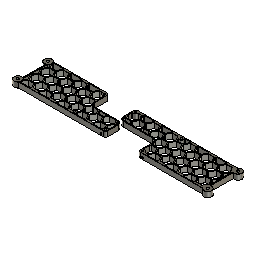
ERCF_Support_Plate_350 (Autodesk Fusion 360 design; units mm, degrees)
Autodesk Fusion 360 part; units mm, degrees
note: some values were not read from the file. Chosen so that the rebuilt part matches the saved one: which pieces of a blend or face edit are solid. Set by a fixed rule: which sketch regions a step uses.
(part 1 of 3)
sketch "Sketch1" plane through (0, 0, 0) normal (0, 0, 1) x (1, 0, 0)
  line L0 (0, 0) -> (490, 0) construction
  line L1 (490, 0) -> (490, 78) construction
  line L2 (490, 78) -> (0, 78) construction
  line L3 (0, 78) -> (0, 0) construction
  circle A0 centre (0, 78) radius 10
  circle A1 centre (0, 0) radius 10
  circle A2 centre (490, 78) radius 10
  circle A3 centre (490, 0) radius 10
  line L4 (0, 39) -> (490, 39) construction
  circle A4 centre (146, 78) radius 2.175
  circle A5 centre (146, 78) radius 6
  line L5 (0, 39) -> (23.382686, 25.5) construction
  line L6 (0, 39) -> (36.373926, 39) construction
  line L7 (23.382686, 25.5) -> (0, 12) construction
  line L8 (23.382686, 25.5) -> (42.918584, 25.5) construction
  line L9 (0, 12) -> (23.382686, -1.5) construction
  line L10 (0, 12) -> (20, 12) construction
  line L11 (220, 78) -> (220, 51.5)
  line L12 (232, 0) -> (232, 26.5)
  line L13 (152, 78) -> (152, 46.5)
  line L14 (316, 31.5) -> (316, 0)
  circle A6 centre (0, 0) radius 3
  circle A7 centre (0, 78) radius 3
  circle A8 centre (490, 0) radius 3
  circle A9 centre (490, 78) radius 3
  line L15 (8, 84) -> (146, 84)
  line L16 (226.000007, 84) -> (482, 84)
  line L17 (482, -6) -> (322.000004, -6)
  line L18 (226, -6) -> (8, -6)
  line L19 (230, 41.5) -> (306, 41.5)
  line L20 (162, 36.5) -> (222, 36.5)
  arc A10 (152, 46.5) -> (162, 36.5) centre (162, 46.5) ccw
  arc A11 (220, 51.5) -> (230, 41.5) centre (230, 51.5) ccw
  arc A12 (316, 31.5) -> (306, 41.5) centre (306, 31.5) ccw
  arc A13 (232, 26.5) -> (222, 36.5) centre (222, 26.5) ccw
  circle A14 centre (146, 0) radius 6
  circle A15 centre (146, 0) radius 2.175
  circle A16 centre (226, 78) radius 6
  circle A17 centre (226, 78) radius 2.175
  circle A18 centre (226, 0) radius 6
  circle A19 centre (226, 0) radius 2.175
  line L21 (149.5, 78) -> (149.5, 46.5)
  arc A20 (149.5, 46.5) -> (162, 34) centre (162, 46.5) ccw
  line L22 (162, 34) -> (222, 34)
  arc A21 (229.5, 26.5) -> (222, 34) centre (222, 26.5) ccw
  line L23 (229.5, 0) -> (229.5, 26.5)
  line L24 (8, 81.5) -> (146, 81.5)
  line L25 (226, -3.5) -> (8, -3.5)
  line L26 (482, -3.5) -> (322.000004, -3.5)
  line L27 (226.000007, 81.5) -> (482, 81.5)
  line L28 (6.928203, 27) -> (13.856406, 39)
  line L29 (13.856406, 39) -> (6.928203, 51)
  line L30 (6.928203, 51) -> (-6.928203, 51)
  line L31 (-6.928203, 51) -> (-13.856406, 39)
  line L32 (-13.856406, 39) -> (-6.928203, 27)
  line L33 (-6.928203, 27) -> (6.928203, 27)
  line L34 (30.310889, 13.5) -> (37.239092, 25.5)
  line L35 (37.239092, 25.5) -> (30.310889, 37.5)
  line L36 (30.310889, 37.5) -> (16.454483, 37.5)
  line L37 (16.454483, 37.5) -> (9.526279, 25.5)
  line L38 (9.526279, 25.5) -> (16.454483, 13.5)
  line L39 (16.454483, 13.5) -> (30.310889, 13.5)
  line L40 (-6.928203, 24) -> (-13.856406, 12)
  line L41 (-13.856406, 12) -> (-6.928203, 0)
  line L42 (-6.928203, 0) -> (6.928203, 0)
  line L43 (6.928203, 0) -> (13.856406, 12)
  line L44 (13.856406, 12) -> (6.928203, 24)
  line L45 (6.928203, 24) -> (-6.928203, 24)
  line L46 (16.454483, 10.5) -> (9.526279, -1.5)
  line L47 (9.526279, -1.5) -> (16.454483, -13.5)
  line L48 (16.454483, -13.5) -> (30.310889, -13.5)
  line L49 (30.310889, -13.5) -> (37.239092, -1.5)
  line L50 (37.239092, -1.5) -> (30.310889, 10.5)
  line L51 (30.310889, 10.5) -> (16.454483, 10.5)
  line L52 (6.928203, 54) -> (13.856406, 66)
  line L53 (13.856406, 66) -> (6.928203, 78)
  line L54 (6.928203, 78) -> (-6.928203, 78)
  line L55 (-6.928203, 78) -> (-13.856406, 66)
  line L56 (-13.856406, 66) -> (-6.928203, 54)
  line L57 (-6.928203, 54) -> (6.928203, 54)
  line L58 (3, 78) -> (3, 0)
  line L59 (487, 78) -> (487, 0)
  line L60 (484, 78) -> (484, 0)
  line L61 (6, 78) -> (6, 0)
  line L62 (222.5, 78) -> (222.5, 51.5)
  arc A22 (222.5, 51.5) -> (230, 44) centre (230, 51.5) ccw
  line L63 (230, 44) -> (306, 44)
  arc A23 (318.5, 31.5) -> (306, 44) centre (306, 31.5) ccw
  line L64 (318.5, 31.5) -> (318.5, 0)
  circle A24 centre (344, 78) radius 2.175
  circle A25 centre (344, 78) radius 6
  circle A26 centre (322, 0) radius 2.175
  circle A27 centre (322, 0) radius 6
  line L65 (32.908965, 12) -> (39.837169, 0)
  line L66 (39.837169, 24) -> (32.908965, 12)
  line L67 (53.693575, 24) -> (39.837169, 24)
  line L68 (60.621778, 12) -> (53.693575, 24)
  line L69 (53.693575, 0) -> (60.621778, 12)
  line L70 (63.219854, 10.5) -> (56.291651, -1.5)
  line L71 (39.837169, 0) -> (53.693575, 0)
  line L72 (53.693575, -3) -> (39.837169, -3)
  line L73 (60.621778, -15) -> (53.693575, -3)
  line L74 (53.693575, -27) -> (60.621778, -15)
  line L75 (39.837169, -27) -> (53.693575, -27)
  line L76 (32.908965, -15) -> (39.837169, -27)
  line L77 (39.837169, -3) -> (32.908965, -15)
  line L78 (77.076261, 10.5) -> (63.219854, 10.5)
  line L79 (56.291651, -1.5) -> (63.219854, -13.5)
  line L80 (63.219854, -13.5) -> (77.076261, -13.5)
  line L81 (77.076261, -13.5) -> (84.004464, -1.5)
  line L82 (84.004464, -1.5) -> (77.076261, 10.5)
  line L83 (77.076261, -16.5) -> (63.219854, -16.5)
  line L84 (63.219854, -16.5) -> (56.291651, -28.5)
  line L85 (56.291651, -28.5) -> (63.219854, -40.5)
  line L86 (63.219854, -40.5) -> (77.076261, -40.5)
  line L87 (77.076261, -40.5) -> (84.004464, -28.5)
  line L88 (84.004464, -28.5) -> (77.076261, -16.5)
  line L89 (79.674337, -15) -> (86.60254, -27)
  line L90 (86.60254, -3) -> (79.674337, -15)
  line L91 (100.458947, -3) -> (86.60254, -3)
  line L92 (107.38715, -15) -> (100.458947, -3)
  line L93 (100.458947, -27) -> (107.38715, -15)
  line L94 (109.985226, -16.5) -> (103.057023, -28.5)
  line L95 (86.60254, -27) -> (100.458947, -27)
  line L96 (100.458947, -30) -> (86.60254, -30)
  line L97 (107.38715, -42) -> (100.458947, -30)
  line L98 (100.458947, -54) -> (107.38715, -42)
  line L99 (86.60254, -54) -> (100.458947, -54)
  line L100 (79.674337, -42) -> (86.60254, -54)
  line L101 (86.60254, -30) -> (79.674337, -42)
  line L102 (123.841633, -16.5) -> (109.985226, -16.5)
  line L103 (103.057023, -28.5) -> (109.985226, -40.5)
  line L104 (109.985226, -40.5) -> (123.841633, -40.5)
  line L105 (123.841633, -40.5) -> (130.769836, -28.5)
  line L106 (130.769836, -28.5) -> (123.841633, -16.5)
  line L107 (123.841633, -43.5) -> (109.985226, -43.5)
  line L108 (109.985226, -43.5) -> (103.057023, -55.5)
  line L109 (103.057023, -55.5) -> (109.985226, -67.5)
  line L110 (109.985226, -67.5) -> (123.841633, -67.5)
  line L111 (123.841633, -67.5) -> (130.769836, -55.5)
  line L112 (130.769836, -55.5) -> (123.841633, -43.5)
  line L113 (126.439709, -42) -> (133.367912, -54)
  line L114 (133.367912, -30) -> (126.439709, -42)
  line L115 (147.224319, -30) -> (133.367912, -30)
  line L116 (154.152522, -42) -> (147.224319, -30)
  line L117 (147.224319, -54) -> (154.152522, -42)
  line L118 (156.750598, -43.5) -> (149.822395, -55.5)
  line L119 (133.367912, -54) -> (147.224319, -54)
  line L120 (147.224319, -57) -> (133.367912, -57)
  line L121 (154.152522, -69) -> (147.224319, -57)
  line L122 (147.224319, -81) -> (154.152522, -69)
  line L123 (133.367912, -81) -> (147.224319, -81)
  line L124 (126.439709, -69) -> (133.367912, -81)
  line L125 (133.367912, -57) -> (126.439709, -69)
  line L126 (170.607005, -43.5) -> (156.750598, -43.5)
  line L127 (149.822395, -55.5) -> (156.750598, -67.5)
  line L128 (156.750598, -67.5) -> (170.607005, -67.5)
  line L129 (170.607005, -67.5) -> (177.535208, -55.5)
  line L130 (177.535208, -55.5) -> (170.607005, -43.5)
  line L131 (170.607005, -70.5) -> (156.750598, -70.5)
  line L132 (156.750598, -70.5) -> (149.822395, -82.5)
  line L133 (149.822395, -82.5) -> (156.750598, -94.5)
  line L134 (156.750598, -94.5) -> (170.607005, -94.5)
  line L135 (170.607005, -94.5) -> (177.535208, -82.5)
  line L136 (177.535208, -82.5) -> (170.607005, -70.5)
  line L137 (173.205081, -69) -> (180.133284, -81)
  line L138 (180.133284, -57) -> (173.205081, -69)
  line L139 (193.98969, -57) -> (180.133284, -57)
  line L140 (200.917894, -69) -> (193.98969, -57)
  line L141 (193.98969, -81) -> (200.917894, -69)
  line L142 (203.51597, -70.5) -> (196.587767, -82.5)
  line L143 (180.133284, -81) -> (193.98969, -81)
  line L144 (193.98969, -84) -> (180.133284, -84)
  line L145 (200.917894, -96) -> (193.98969, -84)
  line L146 (193.98969, -108) -> (200.917894, -96)
  line L147 (180.133284, -108) -> (193.98969, -108)
  line L148 (173.205081, -96) -> (180.133284, -108)
  line L149 (180.133284, -84) -> (173.205081, -96)
  line L150 (217.372376, -70.5) -> (203.51597, -70.5)
  line L151 (196.587767, -82.5) -> (203.51597, -94.5)
  line L152 (203.51597, -94.5) -> (217.372376, -94.5)
  line L153 (217.372376, -94.5) -> (224.30058, -82.5)
  line L154 (224.30058, -82.5) -> (217.372376, -70.5)
  line L155 (217.372376, -97.5) -> (203.51597, -97.5)
  line L156 (203.51597, -97.5) -> (196.587767, -109.5)
  line L157 (196.587767, -109.5) -> (203.51597, -121.5)
  line L158 (203.51597, -121.5) -> (217.372376, -121.5)
  line L159 (217.372376, -121.5) -> (224.30058, -109.5)
  line L160 (224.30058, -109.5) -> (217.372376, -97.5)
  line L161 (219.970453, -96) -> (226.898656, -108)
  line L162 (226.898656, -84) -> (219.970453, -96)
  line L163 (240.755062, -84) -> (226.898656, -84)
  line L164 (247.683265, -96) -> (240.755062, -84)
  line L165 (240.755062, -108) -> (247.683265, -96)
  line L166 (250.281342, -97.5) -> (243.353138, -109.5)
  line L167 (226.898656, -108) -> (240.755062, -108)
  line L168 (240.755062, -111) -> (226.898656, -111)
  line L169 (247.683265, -123) -> (240.755062, -111)
  line L170 (240.755062, -135) -> (247.683265, -123)
  line L171 (226.898656, -135) -> (240.755062, -135)
  line L172 (219.970453, -123) -> (226.898656, -135)
  line L173 (226.898656, -111) -> (219.970453, -123)
  line L174 (264.137748, -97.5) -> (250.281342, -97.5)
  line L175 (243.353138, -109.5) -> (250.281342, -121.5)
  line L176 (250.281342, -121.5) -> (264.137748, -121.5)
  line L177 (264.137748, -121.5) -> (271.065951, -109.5)
  line L178 (271.065951, -109.5) -> (264.137748, -97.5)
  line L179 (264.137748, -124.5) -> (250.281342, -124.5)
  line L180 (250.281342, -124.5) -> (243.353138, -136.5)
  line L181 (243.353138, -136.5) -> (250.281342, -148.5)
  line L182 (250.281342, -148.5) -> (264.137748, -148.5)
  line L183 (264.137748, -148.5) -> (271.065951, -136.5)
  line L184 (271.065951, -136.5) -> (264.137748, -124.5)
  line L185 (266.735824, -123) -> (273.664028, -135)
  line L186 (273.664028, -111) -> (266.735824, -123)
  line L187 (287.520434, -111) -> (273.664028, -111)
  line L188 (294.448637, -123) -> (287.520434, -111)
  line L189 (287.520434, -135) -> (294.448637, -123)
  line L190 (297.046713, -124.5) -> (290.11851, -136.5)
  line L191 (273.664028, -135) -> (287.520434, -135)
  line L192 (287.520434, -138) -> (273.664028, -138)
  line L193 (294.448637, -150) -> (287.520434, -138)
  line L194 (287.520434, -162) -> (294.448637, -150)
  line L195 (273.664028, -162) -> (287.520434, -162)
  line L196 (266.735824, -150) -> (273.664028, -162)
  line L197 (273.664028, -138) -> (266.735824, -150)
  line L198 (310.90312, -124.5) -> (297.046713, -124.5)
  line L199 (290.11851, -136.5) -> (297.046713, -148.5)
  line L200 (297.046713, -148.5) -> (310.90312, -148.5)
  line L201 (310.90312, -148.5) -> (317.831323, -136.5)
  line L202 (317.831323, -136.5) -> (310.90312, -124.5)
  line L203 (310.90312, -151.5) -> (297.046713, -151.5)
  line L204 (297.046713, -151.5) -> (290.11851, -163.5)
  line L205 (290.11851, -163.5) -> (297.046713, -175.5)
  line L206 (297.046713, -175.5) -> (310.90312, -175.5)
  line L207 (310.90312, -175.5) -> (317.831323, -163.5)
  line L208 (317.831323, -163.5) -> (310.90312, -151.5)
  line L209 (313.501196, -150) -> (320.429399, -162)
  line L210 (320.429399, -138) -> (313.501196, -150)
  line L211 (334.285806, -138) -> (320.429399, -138)
  line L212 (341.214009, -150) -> (334.285806, -138)
  line L213 (334.285806, -162) -> (341.214009, -150)
  line L214 (343.812085, -151.5) -> (336.883882, -163.5)
  line L215 (320.429399, -162) -> (334.285806, -162)
  line L216 (334.285806, -165) -> (320.429399, -165)
  line L217 (341.214009, -177) -> (334.285806, -165)
  line L218 (334.285806, -189) -> (341.214009, -177)
  line L219 (320.429399, -189) -> (334.285806, -189)
  line L220 (313.501196, -177) -> (320.429399, -189)
  line L221 (320.429399, -165) -> (313.501196, -177)
  line L222 (357.668492, -151.5) -> (343.812085, -151.5)
  line L223 (336.883882, -163.5) -> (343.812085, -175.5)
  line L224 (343.812085, -175.5) -> (357.668492, -175.5)
  line L225 (357.668492, -175.5) -> (364.596695, -163.5)
  line L226 (364.596695, -163.5) -> (357.668492, -151.5)
  line L227 (357.668492, -178.5) -> (343.812085, -178.5)
  line L228 (343.812085, -178.5) -> (336.883882, -190.5)
  line L229 (336.883882, -190.5) -> (343.812085, -202.5)
  line L230 (343.812085, -202.5) -> (357.668492, -202.5)
  line L231 (357.668492, -202.5) -> (364.596695, -190.5)
  line L232 (364.596695, -190.5) -> (357.668492, -178.5)
  line L233 (360.266568, -177) -> (367.194771, -189)
  line L234 (367.194771, -165) -> (360.266568, -177)
  line L235 (381.051178, -165) -> (367.194771, -165)
  line L236 (387.979381, -177) -> (381.051178, -165)
  line L237 (381.051178, -189) -> (387.979381, -177)
  line L238 (390.577457, -178.5) -> (383.649254, -190.5)
  line L239 (367.194771, -189) -> (381.051178, -189)
  line L240 (381.051178, -192) -> (367.194771, -192)
  line L241 (387.979381, -204) -> (381.051178, -192)
  line L242 (381.051178, -216) -> (387.979381, -204)
  line L243 (367.194771, -216) -> (381.051178, -216)
  line L244 (360.266568, -204) -> (367.194771, -216)
  line L245 (367.194771, -192) -> (360.266568, -204)
  line L246 (404.433864, -178.5) -> (390.577457, -178.5)
  line L247 (383.649254, -190.5) -> (390.577457, -202.5)
  line L248 (390.577457, -202.5) -> (404.433864, -202.5)
  line L249 (404.433864, -202.5) -> (411.362067, -190.5)
  line L250 (411.362067, -190.5) -> (404.433864, -178.5)
  line L251 (404.433864, -205.5) -> (390.577457, -205.5)
  line L252 (390.577457, -205.5) -> (383.649254, -217.5)
  line L253 (383.649254, -217.5) -> (390.577457, -229.5)
  line L254 (390.577457, -229.5) -> (404.433864, -229.5)
  line L255 (404.433864, -229.5) -> (411.362067, -217.5)
  line L256 (411.362067, -217.5) -> (404.433864, -205.5)
  line L257 (9.523594, 79.495348) -> (16.451797, 67.495348)
  line L258 (16.451797, 91.495348) -> (9.523594, 79.495348)
  line L259 (30.308203, 91.495348) -> (16.451797, 91.495348)
  line L260 (37.236406, 79.495348) -> (30.308203, 91.495348)
  line L261 (30.308203, 67.495348) -> (37.236406, 79.495348)
  line L262 (39.834483, 77.995348) -> (32.906279, 65.995348)
  line L263 (16.451797, 67.495348) -> (30.308203, 67.495348)
  line L264 (30.308203, 64.495348) -> (16.451797, 64.495348)
  line L265 (37.236406, 52.495348) -> (30.308203, 64.495348)
  line L266 (30.308203, 40.495348) -> (37.236406, 52.495348)
  line L267 (16.451797, 40.495348) -> (30.308203, 40.495348)
  line L268 (9.523594, 52.495348) -> (16.451797, 40.495348)
  line L269 (16.451797, 64.495348) -> (9.523594, 52.495348)
  line L270 (53.690889, 77.995348) -> (39.834483, 77.995348)
  line L271 (32.906279, 65.995348) -> (39.834483, 53.995348)
  line L272 (39.834483, 53.995348) -> (53.690889, 53.995348)
  line L273 (53.690889, 53.995348) -> (60.619092, 65.995348)
  line L274 (60.619092, 65.995348) -> (53.690889, 77.995348)
  line L275 (53.690889, 50.995348) -> (39.834483, 50.995348)
  line L276 (39.834483, 50.995348) -> (32.906279, 38.995348)
  line L277 (32.906279, 38.995348) -> (39.834483, 26.995348)
  line L278 (39.834483, 26.995348) -> (53.690889, 26.995348)
  line L279 (53.690889, 26.995348) -> (60.619092, 38.995348)
  line L280 (60.619092, 38.995348) -> (53.690889, 50.995348)
  line L281 (56.288965, 52.495348) -> (63.217169, 40.495348)
  line L282 (63.217169, 64.495348) -> (56.288965, 52.495348)
  line L283 (77.073575, 64.495348) -> (63.217169, 64.495348)
  line L284 (84.001778, 52.495348) -> (77.073575, 64.495348)
  line L285 (77.073575, 40.495348) -> (84.001778, 52.495348)
  line L286 (86.599854, 50.995348) -> (79.671651, 38.995348)
  line L287 (63.217169, 40.495348) -> (77.073575, 40.495348)
  line L288 (77.073575, 37.495348) -> (63.217169, 37.495348)
  line L289 (84.001778, 25.495348) -> (77.073575, 37.495348)
  line L290 (77.073575, 13.495348) -> (84.001778, 25.495348)
  line L291 (63.217169, 13.495348) -> (77.073575, 13.495348)
  line L292 (56.288965, 25.495348) -> (63.217169, 13.495348)
  line L293 (63.217169, 37.495348) -> (56.288965, 25.495348)
  line L294 (100.456261, 50.995348) -> (86.599854, 50.995348)
  line L295 (79.671651, 38.995348) -> (86.599854, 26.995348)
  line L296 (86.599854, 26.995348) -> (100.456261, 26.995348)
  line L297 (100.456261, 26.995348) -> (107.384464, 38.995348)
  line L298 (107.384464, 38.995348) -> (100.456261, 50.995348)
  line L299 (100.456261, 23.995348) -> (86.599854, 23.995348)
  line L300 (86.599854, 23.995348) -> (79.671651, 11.995348)
  line L301 (79.671651, 11.995348) -> (86.599854, -0.004652)
  line L302 (86.599854, -0.004652) -> (100.456261, -0.004652)
  line L303 (100.456261, -0.004652) -> (107.384464, 11.995348)
  line L304 (107.384464, 11.995348) -> (100.456261, 23.995348)
  line L305 (103.054337, 25.495348) -> (109.98254, 13.495348)
  line L306 (109.98254, 37.495348) -> (103.054337, 25.495348)
  line L307 (123.838947, 37.495348) -> (109.98254, 37.495348)
  line L308 (130.76715, 25.495348) -> (123.838947, 37.495348)
  line L309 (123.838947, 13.495348) -> (130.76715, 25.495348)
  line L310 (133.365226, 23.995348) -> (126.437023, 11.995348)
  line L311 (109.98254, 13.495348) -> (123.838947, 13.495348)
  line L312 (123.838947, 10.495348) -> (109.98254, 10.495348)
  line L313 (130.76715, -1.504652) -> (123.838947, 10.495348)
  line L314 (123.838947, -13.504652) -> (130.76715, -1.504652)
  line L315 (109.98254, -13.504652) -> (123.838947, -13.504652)
  line L316 (103.054337, -1.504652) -> (109.98254, -13.504652)
  line L317 (109.98254, 10.495348) -> (103.054337, -1.504652)
  line L318 (147.221633, 23.995348) -> (133.365226, 23.995348)
  line L319 (126.437023, 11.995348) -> (133.365226, -0.004652)
  line L320 (133.365226, -0.004652) -> (147.221633, -0.004652)
  line L321 (147.221633, -0.004652) -> (154.149836, 11.995348)
  line L322 (154.149836, 11.995348) -> (147.221633, 23.995348)
  line L323 (147.221633, -3.004652) -> (133.365226, -3.004652)
  line L324 (133.365226, -3.004652) -> (126.437023, -15.004652)
  line L325 (126.437023, -15.004652) -> (133.365226, -27.004652)
  line L326 (133.365226, -27.004652) -> (147.221633, -27.004652)
  line L327 (147.221633, -27.004652) -> (154.149836, -15.004652)
  line L328 (154.149836, -15.004652) -> (147.221633, -3.004652)
  line L329 (149.819709, -1.504652) -> (156.747912, -13.504652)
  line L330 (156.747912, 10.495348) -> (149.819709, -1.504652)
  line L331 (170.604319, 10.495348) -> (156.747912, 10.495348)
  line L332 (177.532522, -1.504652) -> (170.604319, 10.495348)
  line L333 (170.604319, -13.504652) -> (177.532522, -1.504652)
  line L334 (180.130598, -3.004652) -> (173.202395, -15.004652)
  line L335 (156.747912, -13.504652) -> (170.604319, -13.504652)
  line L336 (170.604319, -16.504652) -> (156.747912, -16.504652)
  line L337 (177.532522, -28.504652) -> (170.604319, -16.504652)
  line L338 (170.604319, -40.504652) -> (177.532522, -28.504652)
  line L339 (156.747912, -40.504652) -> (170.604319, -40.504652)
  line L340 (149.819709, -28.504652) -> (156.747912, -40.504652)
  line L341 (156.747912, -16.504652) -> (149.819709, -28.504652)
  line L342 (193.987005, -3.004652) -> (180.130598, -3.004652)
  line L343 (173.202395, -15.004652) -> (180.130598, -27.004652)
  line L344 (180.130598, -27.004652) -> (193.987005, -27.004652)
  line L345 (193.987005, -27.004652) -> (200.915208, -15.004652)
  line L346 (200.915208, -15.004652) -> (193.987005, -3.004652)
  line L347 (193.987005, -30.004652) -> (180.130598, -30.004652)
  line L348 (180.130598, -30.004652) -> (173.202395, -42.004652)
  line L349 (173.202395, -42.004652) -> (180.130598, -54.004652)
  line L350 (180.130598, -54.004652) -> (193.987005, -54.004652)
  line L351 (193.987005, -54.004652) -> (200.915208, -42.004652)
  line L352 (200.915208, -42.004652) -> (193.987005, -30.004652)
  line L353 (196.585081, -28.504652) -> (203.513284, -40.504652)
  line L354 (203.513284, -16.504652) -> (196.585081, -28.504652)
  line L355 (217.36969, -16.504652) -> (203.513284, -16.504652)
  line L356 (224.297894, -28.504652) -> (217.36969, -16.504652)
  line L357 (217.36969, -40.504652) -> (224.297894, -28.504652)
  line L358 (226.89597, -30.004652) -> (219.967767, -42.004652)
  line L359 (203.513284, -40.504652) -> (217.36969, -40.504652)
  line L360 (217.36969, -43.504652) -> (203.513284, -43.504652)
  line L361 (224.297894, -55.504652) -> (217.36969, -43.504652)
  line L362 (217.36969, -67.504652) -> (224.297894, -55.504652)
  line L363 (203.513284, -67.504652) -> (217.36969, -67.504652)
  line L364 (196.585081, -55.504652) -> (203.513284, -67.504652)
  line L365 (203.513284, -43.504652) -> (196.585081, -55.504652)
  line L366 (240.752376, -30.004652) -> (226.89597, -30.004652)
  line L367 (219.967767, -42.004652) -> (226.89597, -54.004652)
  line L368 (226.89597, -54.004652) -> (240.752376, -54.004652)
  line L369 (240.752376, -54.004652) -> (247.68058, -42.004652)
  line L370 (247.68058, -42.004652) -> (240.752376, -30.004652)
  line L371 (240.752376, -57.004652) -> (226.89597, -57.004652)
  line L372 (226.89597, -57.004652) -> (219.967767, -69.004652)
  line L373 (219.967767, -69.004652) -> (226.89597, -81.004652)
  line L374 (226.89597, -81.004652) -> (240.752376, -81.004652)
  line L375 (240.752376, -81.004652) -> (247.68058, -69.004652)
  line L376 (247.68058, -69.004652) -> (240.752376, -57.004652)
  line L377 (243.350453, -55.504652) -> (250.278656, -67.504652)
  line L378 (250.278656, -43.504652) -> (243.350453, -55.504652)
  line L379 (264.135062, -43.504652) -> (250.278656, -43.504652)
  line L380 (271.063265, -55.504652) -> (264.135062, -43.504652)
  line L381 (264.135062, -67.504652) -> (271.063265, -55.504652)
  line L382 (273.661342, -57.004652) -> (266.733138, -69.004652)
  line L383 (250.278656, -67.504652) -> (264.135062, -67.504652)
  line L384 (264.135062, -70.504652) -> (250.278656, -70.504652)
  line L385 (271.063265, -82.504652) -> (264.135062, -70.504652)
  line L386 (264.135062, -94.504652) -> (271.063265, -82.504652)
  line L387 (250.278656, -94.504652) -> (264.135062, -94.504652)
  line L388 (243.350453, -82.504652) -> (250.278656, -94.504652)
  line L389 (250.278656, -70.504652) -> (243.350453, -82.504652)
  line L390 (287.517748, -57.004652) -> (273.661342, -57.004652)
  line L391 (266.733138, -69.004652) -> (273.661342, -81.004652)
  line L392 (273.661342, -81.004652) -> (287.517748, -81.004652)
  line L393 (287.517748, -81.004652) -> (294.445951, -69.004652)
  line L394 (294.445951, -69.004652) -> (287.517748, -57.004652)
  line L395 (287.517748, -84.004652) -> (273.661342, -84.004652)
  line L396 (273.661342, -84.004652) -> (266.733138, -96.004652)
  line L397 (266.733138, -96.004652) -> (273.661342, -108.004652)
  line L398 (273.661342, -108.004652) -> (287.517748, -108.004652)
  line L399 (287.517748, -108.004652) -> (294.445951, -96.004652)
  line L400 (294.445951, -96.004652) -> (287.517748, -84.004652)
  line L401 (290.115824, -82.504652) -> (297.044028, -94.504652)
  line L402 (297.044028, -70.504652) -> (290.115824, -82.504652)
  line L403 (310.900434, -70.504652) -> (297.044028, -70.504652)
  line L404 (317.828637, -82.504652) -> (310.900434, -70.504652)
  line L405 (310.900434, -94.504652) -> (317.828637, -82.504652)
  line L406 (320.426713, -84.004652) -> (313.49851, -96.004652)
  line L407 (297.044028, -94.504652) -> (310.900434, -94.504652)
  line L408 (310.900434, -97.504652) -> (297.044028, -97.504652)
  line L409 (317.828637, -109.504652) -> (310.900434, -97.504652)
  line L410 (310.900434, -121.504652) -> (317.828637, -109.504652)
  line L411 (297.044028, -121.504652) -> (310.900434, -121.504652)
  line L412 (290.115824, -109.504652) -> (297.044028, -121.504652)
  line L413 (297.044028, -97.504652) -> (290.115824, -109.504652)
  line L414 (334.28312, -84.004652) -> (320.426713, -84.004652)
  line L415 (313.49851, -96.004652) -> (320.426713, -108.004652)
  line L416 (320.426713, -108.004652) -> (334.28312, -108.004652)
  line L417 (334.28312, -108.004652) -> (341.211323, -96.004652)
  line L418 (341.211323, -96.004652) -> (334.28312, -84.004652)
  line L419 (334.28312, -111.004652) -> (320.426713, -111.004652)
  line L420 (320.426713, -111.004652) -> (313.49851, -123.004652)
  line L421 (313.49851, -123.004652) -> (320.426713, -135.004652)
  line L422 (320.426713, -135.004652) -> (334.28312, -135.004652)
  line L423 (334.28312, -135.004652) -> (341.211323, -123.004652)
  line L424 (341.211323, -123.004652) -> (334.28312, -111.004652)
  line L425 (336.881196, -109.504652) -> (343.809399, -121.504652)
  line L426 (343.809399, -97.504652) -> (336.881196, -109.504652)
  line L427 (357.665806, -97.504652) -> (343.809399, -97.504652)
  line L428 (364.594009, -109.504652) -> (357.665806, -97.504652)
  line L429 (357.665806, -121.504652) -> (364.594009, -109.504652)
  line L430 (367.192085, -111.004652) -> (360.263882, -123.004652)
  line L431 (343.809399, -121.504652) -> (357.665806, -121.504652)
  line L432 (357.665806, -124.504652) -> (343.809399, -124.504652)
  line L433 (364.594009, -136.504652) -> (357.665806, -124.504652)
  line L434 (357.665806, -148.504652) -> (364.594009, -136.504652)
  line L435 (343.809399, -148.504652) -> (357.665806, -148.504652)
  line L436 (336.881196, -136.504652) -> (343.809399, -148.504652)
  line L437 (343.809399, -124.504652) -> (336.881196, -136.504652)
  line L438 (381.048492, -111.004652) -> (367.192085, -111.004652)
  line L439 (360.263882, -123.004652) -> (367.192085, -135.004652)
  line L440 (367.192085, -135.004652) -> (381.048492, -135.004652)
  line L441 (381.048492, -135.004652) -> (387.976695, -123.004652)
  line L442 (387.976695, -123.004652) -> (381.048492, -111.004652)
  line L443 (381.048492, -138.004652) -> (367.192085, -138.004652)
  line L444 (367.192085, -138.004652) -> (360.263882, -150.004652)
  line L445 (360.263882, -150.004652) -> (367.192085, -162.004652)
  line L446 (367.192085, -162.004652) -> (381.048492, -162.004652)
  line L447 (381.048492, -162.004652) -> (387.976695, -150.004652)
  line L448 (387.976695, -150.004652) -> (381.048492, -138.004652)
  line L449 (383.646568, -136.504652) -> (390.574771, -148.504652)
  line L450 (390.574771, -124.504652) -> (383.646568, -136.504652)
  line L451 (404.431178, -124.504652) -> (390.574771, -124.504652)
  line L452 (411.359381, -136.504652) -> (404.431178, -124.504652)
  line L453 (404.431178, -148.504652) -> (411.359381, -136.504652)
  line L454 (413.957457, -138.004652) -> (407.029254, -150.004652)
  line L455 (390.574771, -148.504652) -> (404.431178, -148.504652)
  line L456 (404.431178, -151.504652) -> (390.574771, -151.504652)
  line L457 (411.359381, -163.504652) -> (404.431178, -151.504652)
  line L458 (404.431178, -175.504652) -> (411.359381, -163.504652)
  line L459 (390.574771, -175.504652) -> (404.431178, -175.504652)
  line L460 (383.646568, -163.504652) -> (390.574771, -175.504652)
  line L461 (390.574771, -151.504652) -> (383.646568, -163.504652)
  line L462 (427.813864, -138.004652) -> (413.957457, -138.004652)
  line L463 (407.029254, -150.004652) -> (413.957457, -162.004652)
  line L464 (413.957457, -162.004652) -> (427.813864, -162.004652)
  line L465 (427.813864, -162.004652) -> (434.742067, -150.004652)
  line L466 (434.742067, -150.004652) -> (427.813864, -138.004652)
  line L467 (427.813864, -165.004652) -> (413.957457, -165.004652)
  line L468 (413.957457, -165.004652) -> (407.029254, -177.004652)
  line L469 (407.029254, -177.004652) -> (413.957457, -189.004652)
  line L470 (413.957457, -189.004652) -> (427.813864, -189.004652)
  line L471 (427.813864, -189.004652) -> (434.742067, -177.004652)
  line L472 (434.742067, -177.004652) -> (427.813864, -165.004652)
  line L473 (32.903594, 119.990696) -> (39.831797, 107.990696)
  line L474 (39.831797, 131.990696) -> (32.903594, 119.990696)
  line L475 (53.688203, 131.990696) -> (39.831797, 131.990696)
  line L476 (60.616406, 119.990696) -> (53.688203, 131.990696)
  line L477 (53.688203, 107.990696) -> (60.616406, 119.990696)
  line L478 (63.214483, 118.490696) -> (56.286279, 106.490696)
  line L479 (39.831797, 107.990696) -> (53.688203, 107.990696)
  line L480 (53.688203, 104.990696) -> (39.831797, 104.990696)
  line L481 (60.616406, 92.990696) -> (53.688203, 104.990696)
  line L482 (53.688203, 80.990696) -> (60.616406, 92.990696)
  line L483 (39.831797, 80.990696) -> (53.688203, 80.990696)
  line L484 (32.903594, 92.990696) -> (39.831797, 80.990696)
  line L485 (39.831797, 104.990696) -> (32.903594, 92.990696)
  line L486 (77.070889, 118.490696) -> (63.214483, 118.490696)
  line L487 (56.286279, 106.490696) -> (63.214483, 94.490696)
  line L488 (63.214483, 94.490696) -> (77.070889, 94.490696)
  line L489 (77.070889, 94.490696) -> (83.999092, 106.490696)
  line L490 (83.999092, 106.490696) -> (77.070889, 118.490696)
  line L491 (77.070889, 91.490696) -> (63.214483, 91.490696)
  line L492 (63.214483, 91.490696) -> (56.286279, 79.490696)
  line L493 (56.286279, 79.490696) -> (63.214483, 67.490696)
  line L494 (63.214483, 67.490696) -> (77.070889, 67.490696)
  line L495 (77.070889, 67.490696) -> (83.999092, 79.490696)
  line L496 (83.999092, 79.490696) -> (77.070889, 91.490696)
  line L497 (79.668965, 92.990696) -> (86.597169, 80.990696)
  line L498 (86.597169, 104.990696) -> (79.668965, 92.990696)
  line L499 (100.453575, 104.990696) -> (86.597169, 104.990696)
  line L500 (107.381778, 92.990696) -> (100.453575, 104.990696)
  line L501 (100.453575, 80.990696) -> (107.381778, 92.990696)
  line L502 (109.979854, 91.490696) -> (103.051651, 79.490696)
  line L503 (86.597169, 80.990696) -> (100.453575, 80.990696)
  line L504 (100.453575, 77.990696) -> (86.597169, 77.990696)
  line L505 (107.381778, 65.990696) -> (100.453575, 77.990696)
  line L506 (100.453575, 53.990696) -> (107.381778, 65.990696)
  line L507 (86.597169, 53.990696) -> (100.453575, 53.990696)
  line L508 (79.668965, 65.990696) -> (86.597169, 53.990696)
  line L509 (86.597169, 77.990696) -> (79.668965, 65.990696)
  line L510 (123.836261, 91.490696) -> (109.979854, 91.490696)
  line L511 (103.051651, 79.490696) -> (109.979854, 67.490696)
  line L512 (109.979854, 67.490696) -> (123.836261, 67.490696)
  line L513 (123.836261, 67.490696) -> (130.764464, 79.490696)
  line L514 (130.764464, 79.490696) -> (123.836261, 91.490696)
  line L515 (123.836261, 64.490696) -> (109.979854, 64.490696)
  line L516 (109.979854, 64.490696) -> (103.051651, 52.490696)
  line L517 (103.051651, 52.490696) -> (109.979854, 40.490696)
  line L518 (109.979854, 40.490696) -> (123.836261, 40.490696)
  line L519 (123.836261, 40.490696) -> (130.764464, 52.490696)
  line L520 (130.764464, 52.490696) -> (123.836261, 64.490696)
  line L521 (126.434337, 65.990696) -> (133.36254, 53.990696)
  line L522 (133.36254, 77.990696) -> (126.434337, 65.990696)
  line L523 (147.218947, 77.990696) -> (133.36254, 77.990696)
  line L524 (154.14715, 65.990696) -> (147.218947, 77.990696)
  line L525 (147.218947, 53.990696) -> (154.14715, 65.990696)
  line L526 (156.745226, 64.490696) -> (149.817023, 52.490696)
  line L527 (133.36254, 53.990696) -> (147.218947, 53.990696)
  line L528 (147.218947, 50.990696) -> (133.36254, 50.990696)
  line L529 (154.14715, 38.990696) -> (147.218947, 50.990696)
  line L530 (147.218947, 26.990696) -> (154.14715, 38.990696)
  line L531 (133.36254, 26.990696) -> (147.218947, 26.990696)
  line L532 (126.434337, 38.990696) -> (133.36254, 26.990696)
  line L533 (133.36254, 50.990696) -> (126.434337, 38.990696)
  line L534 (170.601633, 64.490696) -> (156.745226, 64.490696)
  line L535 (149.817023, 52.490696) -> (156.745226, 40.490696)
  line L536 (156.745226, 40.490696) -> (170.601633, 40.490696)
  line L537 (170.601633, 40.490696) -> (177.529836, 52.490696)
  line L538 (177.529836, 52.490696) -> (170.601633, 64.490696)
  line L539 (170.601633, 37.490696) -> (156.745226, 37.490696)
  line L540 (156.745226, 37.490696) -> (149.817023, 25.490696)
  line L541 (149.817023, 25.490696) -> (156.745226, 13.490696)
  line L542 (156.745226, 13.490696) -> (170.601633, 13.490696)
  line L543 (170.601633, 13.490696) -> (177.529836, 25.490696)
  line L544 (177.529836, 25.490696) -> (170.601633, 37.490696)
  line L545 (173.199709, 38.990696) -> (180.127912, 26.990696)
  line L546 (180.127912, 50.990696) -> (173.199709, 38.990696)
  line L547 (193.984319, 50.990696) -> (180.127912, 50.990696)
  line L548 (200.912522, 38.990696) -> (193.984319, 50.990696)
  line L549 (193.984319, 26.990696) -> (200.912522, 38.990696)
  line L550 (203.510598, 37.490696) -> (196.582395, 25.490696)
  line L551 (180.127912, 26.990696) -> (193.984319, 26.990696)
  line L552 (193.984319, 23.990696) -> (180.127912, 23.990696)
  line L553 (200.912522, 11.990696) -> (193.984319, 23.990696)
  line L554 (193.984319, -0.009304) -> (200.912522, 11.990696)
  line L555 (180.127912, -0.009304) -> (193.984319, -0.009304)
  line L556 (173.199709, 11.990696) -> (180.127912, -0.009304)
  line L557 (180.127912, 23.990696) -> (173.199709, 11.990696)
  line L558 (217.367005, 37.490696) -> (203.510598, 37.490696)
  line L559 (196.582395, 25.490696) -> (203.510598, 13.490696)
  line L560 (203.510598, 13.490696) -> (217.367005, 13.490696)
  line L561 (217.367005, 13.490696) -> (224.295208, 25.490696)
  line L562 (224.295208, 25.490696) -> (217.367005, 37.490696)
  line L563 (217.367005, 10.490696) -> (203.510598, 10.490696)
  line L564 (203.510598, 10.490696) -> (196.582395, -1.509304)
  line L565 (196.582395, -1.509304) -> (203.510598, -13.509304)
  line L566 (203.510598, -13.509304) -> (217.367005, -13.509304)
  line L567 (217.367005, -13.509304) -> (224.295208, -1.509304)
  line L568 (224.295208, -1.509304) -> (217.367005, 10.490696)
  line L569 (219.965081, 11.990696) -> (226.893284, -0.009304)
  line L570 (226.893284, 23.990696) -> (219.965081, 11.990696)
  line L571 (240.74969, 23.990696) -> (226.893284, 23.990696)
  line L572 (247.677894, 11.990696) -> (240.74969, 23.990696)
  line L573 (240.74969, -0.009304) -> (247.677894, 11.990696)
  line L574 (250.27597, 10.490696) -> (243.347767, -1.509304)
  line L575 (226.893284, -0.009304) -> (240.74969, -0.009304)
  line L576 (240.74969, -3.009304) -> (226.893284, -3.009304)
  line L577 (247.677894, -15.009304) -> (240.74969, -3.009304)
  line L578 (240.74969, -27.009304) -> (247.677894, -15.009304)
  line L579 (226.893284, -27.009304) -> (240.74969, -27.009304)
  line L580 (219.965081, -15.009304) -> (226.893284, -27.009304)
  line L581 (226.893284, -3.009304) -> (219.965081, -15.009304)
  line L582 (264.132376, 10.490696) -> (250.27597, 10.490696)
  line L583 (243.347767, -1.509304) -> (250.27597, -13.509304)
  line L584 (250.27597, -13.509304) -> (264.132376, -13.509304)
  line L585 (264.132376, -13.509304) -> (271.06058, -1.509304)
  line L586 (271.06058, -1.509304) -> (264.132376, 10.490696)
  line L587 (264.132376, -16.509304) -> (250.27597, -16.509304)
  line L588 (250.27597, -16.509304) -> (243.347767, -28.509304)
  line L589 (243.347767, -28.509304) -> (250.27597, -40.509304)
  line L590 (250.27597, -40.509304) -> (264.132376, -40.509304)
  line L591 (264.132376, -40.509304) -> (271.06058, -28.509304)
  line L592 (271.06058, -28.509304) -> (264.132376, -16.509304)
  line L593 (266.730453, -15.009304) -> (273.658656, -27.009304)
  line L594 (273.658656, -3.009304) -> (266.730453, -15.009304)
  line L595 (287.515062, -3.009304) -> (273.658656, -3.009304)
  line L596 (294.443265, -15.009304) -> (287.515062, -3.009304)
  line L597 (287.515062, -27.009304) -> (294.443265, -15.009304)
  line L598 (297.041342, -16.509304) -> (290.113138, -28.509304)
  line L599 (273.658656, -27.009304) -> (287.515062, -27.009304)
  line L600 (287.515062, -30.009304) -> (273.658656, -30.009304)
  line L601 (294.443265, -42.009304) -> (287.515062, -30.009304)
  line L602 (287.515062, -54.009304) -> (294.443265, -42.009304)
  line L603 (273.658656, -54.009304) -> (287.515062, -54.009304)
  line L604 (266.730453, -42.009304) -> (273.658656, -54.009304)
  line L605 (273.658656, -30.009304) -> (266.730453, -42.009304)
  line L606 (310.897748, -16.509304) -> (297.041342, -16.509304)
  line L607 (290.113138, -28.509304) -> (297.041342, -40.509304)
  line L608 (297.041342, -40.509304) -> (310.897748, -40.509304)
  line L609 (310.897748, -40.509304) -> (317.825951, -28.509304)
  line L610 (317.825951, -28.509304) -> (310.897748, -16.509304)
  line L611 (310.897748, -43.509304) -> (297.041342, -43.509304)
  line L612 (297.041342, -43.509304) -> (290.113138, -55.509304)
  line L613 (290.113138, -55.509304) -> (297.041342, -67.509304)
  line L614 (297.041342, -67.509304) -> (310.897748, -67.509304)
  line L615 (310.897748, -67.509304) -> (317.825951, -55.509304)
  line L616 (317.825951, -55.509304) -> (310.897748, -43.509304)
  line L617 (313.495824, -42.009304) -> (320.424028, -54.009304)
  line L618 (320.424028, -30.009304) -> (313.495824, -42.009304)
  line L619 (334.280434, -30.009304) -> (320.424028, -30.009304)
  line L620 (341.208637, -42.009304) -> (334.280434, -30.009304)
  line L621 (334.280434, -54.009304) -> (341.208637, -42.009304)
  line L622 (343.806713, -43.509304) -> (336.87851, -55.509304)
  line L623 (320.424028, -54.009304) -> (334.280434, -54.009304)
  line L624 (334.280434, -57.009304) -> (320.424028, -57.009304)
  line L625 (341.208637, -69.009304) -> (334.280434, -57.009304)
  line L626 (334.280434, -81.009304) -> (341.208637, -69.009304)
  line L627 (320.424028, -81.009304) -> (334.280434, -81.009304)
  line L628 (313.495824, -69.009304) -> (320.424028, -81.009304)
  line L629 (320.424028, -57.009304) -> (313.495824, -69.009304)
  line L630 (357.66312, -43.509304) -> (343.806713, -43.509304)
  line L631 (336.87851, -55.509304) -> (343.806713, -67.509304)
  line L632 (343.806713, -67.509304) -> (357.66312, -67.509304)
  line L633 (357.66312, -67.509304) -> (364.591323, -55.509304)
  line L634 (364.591323, -55.509304) -> (357.66312, -43.509304)
  line L635 (357.66312, -70.509304) -> (343.806713, -70.509304)
  line L636 (343.806713, -70.509304) -> (336.87851, -82.509304)
  line L637 (336.87851, -82.509304) -> (343.806713, -94.509304)
  line L638 (343.806713, -94.509304) -> (357.66312, -94.509304)
  line L639 (357.66312, -94.509304) -> (364.591323, -82.509304)
  line L640 (364.591323, -82.509304) -> (357.66312, -70.509304)
  line L641 (360.261196, -69.009304) -> (367.189399, -81.009304)
  line L642 (367.189399, -57.009304) -> (360.261196, -69.009304)
  line L643 (381.045806, -57.009304) -> (367.189399, -57.009304)
  line L644 (387.974009, -69.009304) -> (381.045806, -57.009304)
  line L645 (381.045806, -81.009304) -> (387.974009, -69.009304)
  line L646 (390.572085, -70.509304) -> (383.643882, -82.509304)
  line L647 (367.189399, -81.009304) -> (381.045806, -81.009304)
  line L648 (381.045806, -84.009304) -> (367.189399, -84.009304)
  line L649 (387.974009, -96.009304) -> (381.045806, -84.009304)
  line L650 (381.045806, -108.009304) -> (387.974009, -96.009304)
  line L651 (367.189399, -108.009304) -> (381.045806, -108.009304)
  line L652 (360.261196, -96.009304) -> (367.189399, -108.009304)
  line L653 (367.189399, -84.009304) -> (360.261196, -96.009304)
  line L654 (404.428492, -70.509304) -> (390.572085, -70.509304)
  line L655 (383.643882, -82.509304) -> (390.572085, -94.509304)
  line L656 (390.572085, -94.509304) -> (404.428492, -94.509304)
  line L657 (404.428492, -94.509304) -> (411.356695, -82.509304)
  line L658 (411.356695, -82.509304) -> (404.428492, -70.509304)
  line L659 (404.428492, -97.509304) -> (390.572085, -97.509304)
  line L660 (390.572085, -97.509304) -> (383.643882, -109.509304)
  line L661 (383.643882, -109.509304) -> (390.572085, -121.509304)
  line L662 (390.572085, -121.509304) -> (404.428492, -121.509304)
  line L663 (404.428492, -121.509304) -> (411.356695, -109.509304)
  line L664 (411.356695, -109.509304) -> (404.428492, -97.509304)
  line L665 (407.026568, -96.009304) -> (413.954771, -108.009304)
  line L666 (413.954771, -84.009304) -> (407.026568, -96.009304)
  line L667 (427.811178, -84.009304) -> (413.954771, -84.009304)
  line L668 (434.739381, -96.009304) -> (427.811178, -84.009304)
  line L669 (427.811178, -108.009304) -> (434.739381, -96.009304)
  line L670 (437.337457, -97.509304) -> (430.409254, -109.509304)
  line L671 (413.954771, -108.009304) -> (427.811178, -108.009304)
  line L672 (427.811178, -111.009304) -> (413.954771, -111.009304)
  line L673 (434.739381, -123.009304) -> (427.811178, -111.009304)
  line L674 (427.811178, -135.009304) -> (434.739381, -123.009304)
  line L675 (413.954771, -135.009304) -> (427.811178, -135.009304)
  line L676 (407.026568, -123.009304) -> (413.954771, -135.009304)
  line L677 (413.954771, -111.009304) -> (407.026568, -123.009304)
  line L678 (451.193864, -97.509304) -> (437.337457, -97.509304)
  line L679 (430.409254, -109.509304) -> (437.337457, -121.509304)
  line L680 (437.337457, -121.509304) -> (451.193864, -121.509304)
  line L681 (451.193864, -121.509304) -> (458.122067, -109.509304)
  line L682 (458.122067, -109.509304) -> (451.193864, -97.509304)
  line L683 (451.193864, -124.509304) -> (437.337457, -124.509304)
  line L684 (437.337457, -124.509304) -> (430.409254, -136.509304)
  line L685 (430.409254, -136.509304) -> (437.337457, -148.509304)
  line L686 (437.337457, -148.509304) -> (451.193864, -148.509304)
  line L687 (451.193864, -148.509304) -> (458.122067, -136.509304)
  line L688 (458.122067, -136.509304) -> (451.193864, -124.509304)
  line L689 (56.283594, 160.486044) -> (63.211797, 148.486044)
  line L690 (63.211797, 172.486044) -> (56.283594, 160.486044)
  line L691 (77.068203, 172.486044) -> (63.211797, 172.486044)
  line L692 (83.996406, 160.486044) -> (77.068203, 172.486044)
  line L693 (77.068203, 148.486044) -> (83.996406, 160.486044)
  line L694 (86.594483, 158.986044) -> (79.666279, 146.986044)
  line L695 (63.211797, 148.486044) -> (77.068203, 148.486044)
  line L696 (77.068203, 145.486044) -> (63.211797, 145.486044)
  line L697 (83.996406, 133.486044) -> (77.068203, 145.486044)
  line L698 (77.068203, 121.486044) -> (83.996406, 133.486044)
  line L699 (63.211797, 121.486044) -> (77.068203, 121.486044)
  line L700 (56.283594, 133.486044) -> (63.211797, 121.486044)
  line L701 (63.211797, 145.486044) -> (56.283594, 133.486044)
  line L702 (100.450889, 158.986044) -> (86.594483, 158.986044)
  line L703 (79.666279, 146.986044) -> (86.594483, 134.986044)
  line L704 (86.594483, 134.986044) -> (100.450889, 134.986044)
  line L705 (100.450889, 134.986044) -> (107.379092, 146.986044)
  line L706 (107.379092, 146.986044) -> (100.450889, 158.986044)
  line L707 (100.450889, 131.986044) -> (86.594483, 131.986044)
  line L708 (86.594483, 131.986044) -> (79.666279, 119.986044)
  line L709 (79.666279, 119.986044) -> (86.594483, 107.986044)
  line L710 (86.594483, 107.986044) -> (100.450889, 107.986044)
  line L711 (100.450889, 107.986044) -> (107.379092, 119.986044)
  line L712 (107.379092, 119.986044) -> (100.450889, 131.986044)
  line L713 (103.048965, 133.486044) -> (109.977169, 121.486044)
  line L714 (109.977169, 145.486044) -> (103.048965, 133.486044)
  line L715 (123.833575, 145.486044) -> (109.977169, 145.486044)
  line L716 (130.761778, 133.486044) -> (123.833575, 145.486044)
  line L717 (123.833575, 121.486044) -> (130.761778, 133.486044)
  line L718 (133.359854, 131.986044) -> (126.431651, 119.986044)
  line L719 (109.977169, 121.486044) -> (123.833575, 121.486044)
  line L720 (123.833575, 118.486044) -> (109.977169, 118.486044)
  line L721 (130.761778, 106.486044) -> (123.833575, 118.486044)
  line L722 (123.833575, 94.486044) -> (130.761778, 106.486044)
  line L723 (109.977169, 94.486044) -> (123.833575, 94.486044)
  line L724 (103.048965, 106.486044) -> (109.977169, 94.486044)
  line L725 (109.977169, 118.486044) -> (103.048965, 106.486044)
  line L726 (147.216261, 131.986044) -> (133.359854, 131.986044)
  line L727 (126.431651, 119.986044) -> (133.359854, 107.986044)
  line L728 (133.359854, 107.986044) -> (147.216261, 107.986044)
  line L729 (147.216261, 107.986044) -> (154.144464, 119.986044)
  line L730 (154.144464, 119.986044) -> (147.216261, 131.986044)
  line L731 (147.216261, 104.986044) -> (133.359854, 104.986044)
  line L732 (133.359854, 104.986044) -> (126.431651, 92.986044)
  line L733 (126.431651, 92.986044) -> (133.359854, 80.986044)
  line L734 (133.359854, 80.986044) -> (147.216261, 80.986044)
  line L735 (147.216261, 80.986044) -> (154.144464, 92.986044)
  line L736 (154.144464, 92.986044) -> (147.216261, 104.986044)
  line L737 (149.814337, 106.486044) -> (156.74254, 94.486044)
  line L738 (156.74254, 118.486044) -> (149.814337, 106.486044)
  line L739 (170.598947, 118.486044) -> (156.74254, 118.486044)
  line L740 (177.52715, 106.486044) -> (170.598947, 118.486044)
  line L741 (170.598947, 94.486044) -> (177.52715, 106.486044)
  line L742 (180.125226, 104.986044) -> (173.197023, 92.986044)
  line L743 (156.74254, 94.486044) -> (170.598947, 94.486044)
  line L744 (170.598947, 91.486044) -> (156.74254, 91.486044)
  line L745 (177.52715, 79.486044) -> (170.598947, 91.486044)
  line L746 (170.598947, 67.486044) -> (177.52715, 79.486044)
  line L747 (156.74254, 67.486044) -> (170.598947, 67.486044)
  line L748 (149.814337, 79.486044) -> (156.74254, 67.486044)
  line L749 (156.74254, 91.486044) -> (149.814337, 79.486044)
  line L750 (193.981633, 104.986044) -> (180.125226, 104.986044)
  line L751 (173.197023, 92.986044) -> (180.125226, 80.986044)
  line L752 (180.125226, 80.986044) -> (193.981633, 80.986044)
  line L753 (193.981633, 80.986044) -> (200.909836, 92.986044)
  line L754 (200.909836, 92.986044) -> (193.981633, 104.986044)
  line L755 (193.981633, 77.986044) -> (180.125226, 77.986044)
  line L756 (180.125226, 77.986044) -> (173.197023, 65.986044)
  line L757 (173.197023, 65.986044) -> (180.125226, 53.986044)
  line L758 (180.125226, 53.986044) -> (193.981633, 53.986044)
  line L759 (193.981633, 53.986044) -> (200.909836, 65.986044)
  line L760 (200.909836, 65.986044) -> (193.981633, 77.986044)
  line L761 (196.579709, 79.486044) -> (203.507912, 67.486044)
  line L762 (203.507912, 91.486044) -> (196.579709, 79.486044)
  line L763 (217.364319, 91.486044) -> (203.507912, 91.486044)
  line L764 (224.292522, 79.486044) -> (217.364319, 91.486044)
  line L765 (217.364319, 67.486044) -> (224.292522, 79.486044)
  line L766 (226.890598, 77.986044) -> (219.962395, 65.986044)
  line L767 (203.507912, 67.486044) -> (217.364319, 67.486044)
  line L768 (217.364319, 64.486044) -> (203.507912, 64.486044)
  line L769 (224.292522, 52.486044) -> (217.364319, 64.486044)
  line L770 (217.364319, 40.486044) -> (224.292522, 52.486044)
  line L771 (203.507912, 40.486044) -> (217.364319, 40.486044)
  line L772 (196.579709, 52.486044) -> (203.507912, 40.486044)
  line L773 (203.507912, 64.486044) -> (196.579709, 52.486044)
  line L774 (240.747005, 77.986044) -> (226.890598, 77.986044)
  line L775 (219.962395, 65.986044) -> (226.890598, 53.986044)
  line L776 (226.890598, 53.986044) -> (240.747005, 53.986044)
  line L777 (240.747005, 53.986044) -> (247.675208, 65.986044)
  line L778 (247.675208, 65.986044) -> (240.747005, 77.986044)
  line L779 (240.747005, 50.986044) -> (226.890598, 50.986044)
  line L780 (226.890598, 50.986044) -> (219.962395, 38.986044)
  line L781 (219.962395, 38.986044) -> (226.890598, 26.986044)
  line L782 (226.890598, 26.986044) -> (240.747005, 26.986044)
  line L783 (240.747005, 26.986044) -> (247.675208, 38.986044)
  line L784 (247.675208, 38.986044) -> (240.747005, 50.986044)
  line L785 (243.345081, 52.486044) -> (250.273284, 40.486044)
  line L786 (250.273284, 64.486044) -> (243.345081, 52.486044)
  line L787 (264.12969, 64.486044) -> (250.273284, 64.486044)
  line L788 (271.057894, 52.486044) -> (264.12969, 64.486044)
  line L789 (264.12969, 40.486044) -> (271.057894, 52.486044)
  line L790 (273.65597, 50.986044) -> (266.727767, 38.986044)
  line L791 (250.273284, 40.486044) -> (264.12969, 40.486044)
  line L792 (264.12969, 37.486044) -> (250.273284, 37.486044)
  line L793 (271.057894, 25.486044) -> (264.12969, 37.486044)
  line L794 (264.12969, 13.486044) -> (271.057894, 25.486044)
  line L795 (250.273284, 13.486044) -> (264.12969, 13.486044)
  line L796 (243.345081, 25.486044) -> (250.273284, 13.486044)
  line L797 (250.273284, 37.486044) -> (243.345081, 25.486044)
  line L798 (287.512376, 50.986044) -> (273.65597, 50.986044)
  line L799 (266.727767, 38.986044) -> (273.65597, 26.986044)
  line L800 (273.65597, 26.986044) -> (287.512376, 26.986044)
  line L801 (287.512376, 26.986044) -> (294.44058, 38.986044)
  line L802 (294.44058, 38.986044) -> (287.512376, 50.986044)
  line L803 (287.512376, 23.986044) -> (273.65597, 23.986044)
  line L804 (273.65597, 23.986044) -> (266.727767, 11.986044)